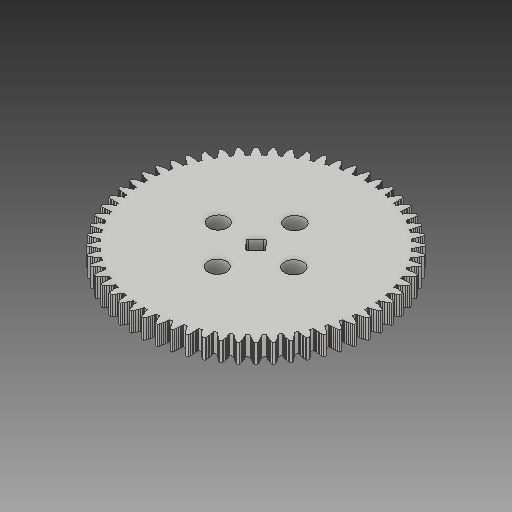
# Autodesk Inventor part: gear60
Saved by Autodesk Inventor 2019 (Build 230136000, 136)
## iProperties
Created: 2019-01-24
Part Number: gear60
Material: Generic
Document SubType Name: Modeling
Designer: Varga Daniel
Density: 1 g/cm^3
Appearance: Default
Author: Varga Daniel
Autodesk Inventor part; units mm, degrees
(part 1 of 2)
ref_plane "YZ Plane" through (0, 0, 0) normal (1, 0, 0) x (0, 1, 0)
ref_plane "XZ Plane" through (0, 0, 0) normal (0, 1, 0) x (-1, 0, 0)
ref_plane "XY Plane" through (0, 0, 0) normal (0, 0, 1) x (1, 0, 0)
sketch "Sketch7" plane through (0, 0, 0) normal (0, 1, 0) x (-1, 0, 0)
  line L0 (2.4527, 31.6296) -> (2.3509, 31.6528)
  line L1 (2.3509, 31.6528) -> (2.2492, 31.6779)
  line L2 (2.2492, 31.6779) -> (2.0459, 31.7329)
  line L3 (2.0459, 31.7329) -> (1.64, 31.8609)
  line L4 (1.64, 31.8609) -> (1.2352, 32.0102)
  line L5 (1.2352, 32.0102) -> (0.8316, 32.1789)
  line L6 (0.8316, 32.1789) -> (0.4294, 32.3655)
  line L7 (0.4294, 32.3655) -> (0.0289, 32.5691)
  line L8 (0.0289, 32.5691) -> (0.0593, 33.1489)
  line L9 (0.0593, 33.1489) -> (0.4789, 33.3096)
  line L10 (0.4789, 33.3096) -> (0.8983, 33.4531)
  line L11 (0.8983, 33.4531) -> (1.3174, 33.5787)
  line L12 (1.3174, 33.5787) -> (1.7356, 33.6849)
  line L13 (1.7356, 33.6849) -> (2.1527, 33.7697)
  line L14 (2.1527, 33.7697) -> (2.3606, 33.8032)
  line L15 (2.3606, 33.8032) -> (2.4644, 33.8175)
  line L16 (2.4644, 33.8175) -> (2.568, 33.83)
  line L17 (2.568, 33.83) -> (2.6526, 34.6349)
  line L18 (2.6526, 34.6349) -> (2.5538, 34.6686)
  line L19 (2.5538, 34.6686) -> (2.4553, 34.7042)
  line L20 (2.4553, 34.7042) -> (2.2589, 34.7802)
  line L21 (2.2589, 34.7802) -> (1.8686, 34.9499)
  line L22 (1.8686, 34.9499) -> (1.4816, 35.1407)
  line L23 (1.4816, 35.1407) -> (1.0978, 35.3506)
  line L24 (1.0978, 35.3506) -> (0.7173, 35.5783)
  line L25 (0.7173, 35.5783) -> (0.3404, 35.8226)
  line L26 (0.3404, 35.8226) -> (0.4312, 36.3961)
  line L27 (0.4312, 36.3961) -> (0.8652, 36.512)
  line L28 (0.8652, 36.512) -> (1.2974, 36.6109)
  line L29 (1.2974, 36.6109) -> (1.7273, 36.692)
  line L30 (1.7273, 36.692) -> (2.1543, 36.7538)
  line L31 (2.1543, 36.7538) -> (2.5779, 36.7946)
  line L32 (2.5779, 36.7946) -> (2.7882, 36.8062)
  line L33 (2.7882, 36.8062) -> (2.8929, 36.8096)
  line L34 (2.8929, 36.8096) -> (2.9973, 36.8112)
  line L35 (2.9973, 36.8112) -> (3.1655, 37.6028)
  line L36 (3.1655, 37.6028) -> (3.0708, 37.6467)
  line L37 (3.0708, 37.6467) -> (2.9766, 37.6924)
  line L38 (2.9766, 37.6924) -> (2.7892, 37.7885)
  line L39 (2.7892, 37.7885) -> (2.4188, 37.998)
  line L40 (2.4188, 37.998) -> (2.0538, 38.2283)
  line L41 (2.0538, 38.2283) -> (1.6941, 38.4772)
  line L42 (1.6941, 38.4772) -> (1.3395, 38.7433)
  line L43 (1.3395, 38.7433) -> (0.9901, 39.0258)
  line L44 (0.9901, 39.0258) -> (1.1404, 39.5866)
  line L45 (1.1404, 39.5866) -> (1.5842, 39.6565)
  line L46 (1.5842, 39.6565) -> (2.0243, 39.7097)
  line L47 (2.0243, 39.7097) -> (2.4603, 39.7454)
  line L48 (2.4603, 39.7454) -> (2.8915, 39.7623)
  line L49 (2.8915, 39.7623) -> (3.3171, 39.7586)
  line L50 (3.3171, 39.7586) -> (3.5274, 39.7481)
  line L51 (3.5274, 39.7481) -> (3.6319, 39.7405)
  line L52 (3.6319, 39.7405) -> (3.7358, 39.7312)
  line L53 (3.7358, 39.7312) -> (3.9859, 40.5009)
  line L54 (3.9859, 40.5009) -> (3.8963, 40.5544)
  line L55 (3.8963, 40.5544) -> (3.8074, 40.6097)
  line L56 (3.8074, 40.6097) -> (3.631, 40.7249)
  line L57 (3.631, 40.7249) -> (3.2846, 40.972)
  line L58 (3.2846, 40.972) -> (2.9457, 41.2391)
  line L59 (2.9457, 41.2391) -> (2.6139, 41.5242)
  line L60 (2.6139, 41.5242) -> (2.2891, 41.826)
  line L61 (2.2891, 41.826) -> (1.9712, 42.1434)
  line L62 (1.9712, 42.1434) -> (2.1792, 42.6854)
  line L63 (2.1792, 42.6854) -> (2.6279, 42.7086)
  line L64 (2.6279, 42.7086) -> (3.0712, 42.7155)
  line L65 (3.0712, 42.7155) -> (3.5085, 42.7054)
  line L66 (3.5085, 42.7054) -> (3.9391, 42.6771)
  line L67 (3.9391, 42.6771) -> (4.362, 42.629)
  line L68 (4.362, 42.629) -> (4.5701, 42.5966)
  line L69 (4.5701, 42.5966) -> (4.6731, 42.5781)
  line L70 (4.6731, 42.5781) -> (4.7756, 42.558)
  line L71 (4.7756, 42.558) -> (5.1047, 43.2973)
  line L72 (5.1047, 43.2973) -> (5.0212, 43.3599)
  line L73 (5.0212, 43.3599) -> (4.9385, 43.4242)
  line L74 (4.9385, 43.4242) -> (4.7752, 43.5572)
  line L75 (4.7752, 43.5572) -> (4.4565, 43.8392)
  line L76 (4.4565, 43.8392) -> (4.1474, 44.1402)
  line L77 (4.1474, 44.1402) -> (3.8472, 44.4585)
  line L78 (3.8472, 44.4585) -> (3.5558, 44.7925)
  line L79 (3.5558, 44.7925) -> (3.2727, 45.1414)
  line L80 (3.2727, 45.1414) -> (3.5363, 45.6588)
  line L81 (3.5363, 45.6588) -> (3.9849, 45.6349)
  line L82 (3.9849, 45.6349) -> (4.4265, 45.5954)
  line L83 (4.4265, 45.5954) -> (4.8604, 45.5397)
  line L84 (4.8604, 45.5397) -> (5.2857, 45.4666)
  line L85 (5.2857, 45.4666) -> (5.7012, 45.3744)
  line L86 (5.7012, 45.3744) -> (5.9047, 45.3205)
  line L87 (5.9047, 45.3205) -> (6.0053, 45.2913)
  line L88 (6.0053, 45.2913) -> (6.1051, 45.2606)
  line L89 (6.1051, 45.2606) -> (6.5097, 45.9615)
  line L90 (6.5097, 45.9615) -> (6.4333, 46.0325)
  line L91 (6.4333, 46.0325) -> (6.3577, 46.105)
  line L92 (6.3577, 46.105) -> (6.2092, 46.2543)
  line L93 (6.2092, 46.2543) -> (5.9217, 46.5681)
  line L94 (5.9217, 46.5681) -> (5.6457, 46.8999)
  line L95 (5.6457, 46.8999) -> (5.3805, 47.2477)
  line L96 (5.3805, 47.2477) -> (5.1255, 47.6104)
  line L97 (5.1255, 47.6104) -> (4.8805, 47.987)
  line L98 (4.8805, 47.987) -> (5.1967, 48.4739)
  line L99 (5.1967, 48.4739) -> (5.6404, 48.4033)
  line L100 (5.6404, 48.4033) -> (6.0755, 48.3179)
  line L101 (6.0755, 48.3179) -> (6.5011, 48.2171)
  line L102 (6.5011, 48.2171) -> (6.9164, 48.0999)
  line L103 (6.9164, 48.0999) -> (7.32, 47.9649)
  line L104 (7.32, 47.9649) -> (7.5168, 47.8899)
  line L105 (7.5168, 47.8899) -> (7.6138, 47.8504)
  line L106 (7.6138, 47.8504) -> (7.7098, 47.8094)
  line L107 (7.7098, 47.8094) -> (8.1855, 48.4642)
  line L108 (8.1855, 48.4642) -> (8.1169, 48.5428)
  line L109 (8.1169, 48.5428) -> (8.0493, 48.6228)
  line L110 (8.0493, 48.6228) -> (7.9172, 48.7869)
  line L111 (7.9172, 48.7869) -> (7.6641, 49.129)
  line L112 (7.6641, 49.129) -> (7.4243, 49.4878)
  line L113 (7.4243, 49.4878) -> (7.1969, 49.8614)
  line L114 (7.1969, 49.8614) -> (6.9813, 50.2488)
  line L115 (6.9813, 50.2488) -> (6.777, 50.6489)
  line L116 (6.777, 50.6489) -> (7.1423, 51.1001)
  line L117 (7.1423, 51.1001) -> (7.5762, 50.9835)
  line L118 (7.5762, 50.9835) -> (7.9999, 50.8531)
  line L119 (7.9999, 50.8531) -> (8.4127, 50.7084)
  line L120 (8.4127, 50.7084) -> (8.8135, 50.5484)
  line L121 (8.8135, 50.5484) -> (9.2008, 50.3719)
  line L122 (9.2008, 50.3719) -> (9.3887, 50.2768)
  line L123 (9.3887, 50.2768) -> (9.481, 50.2274)
  line L124 (9.481, 50.2274) -> (9.5722, 50.1766)
  line L125 (9.5722, 50.1766) -> (10.1137, 50.778)
  line L126 (10.1137, 50.778) -> (10.0537, 50.8634)
  line L127 (10.0537, 50.8634) -> (9.9948, 50.9501)
  line L128 (9.9948, 50.9501) -> (9.8806, 51.127)
  line L129 (9.8806, 51.127) -> (9.6646, 51.4937)
  line L130 (9.6646, 51.4937) -> (9.4637, 51.8755)
  line L131 (9.4637, 51.8755) -> (9.2766, 52.2709)
  line L132 (9.2766, 52.2709) -> (9.1026, 52.6787)
  line L133 (9.1026, 52.6787) -> (8.9413, 53.098)
  line L134 (8.9413, 53.098) -> (9.3518, 53.5086)
  line L135 (9.3518, 53.5086) -> (9.7711, 53.3472)
  line L136 (9.7711, 53.3472) -> (10.1789, 53.1732)
  line L137 (10.1789, 53.1732) -> (10.5743, 52.9861)
  line L138 (10.5743, 52.9861) -> (10.9561, 52.7852)
  line L139 (10.9561, 52.7852) -> (11.3228, 52.5692)
  line L140 (11.3228, 52.5692) -> (11.4998, 52.455)
  line L141 (11.4998, 52.455) -> (11.5864, 52.3961)
  line L142 (11.5864, 52.3961) -> (11.6718, 52.3361)
  line L143 (11.6718, 52.3361) -> (12.2732, 52.8776)
  line L144 (12.2732, 52.8776) -> (12.2224, 52.9688)
  line L145 (12.2224, 52.9688) -> (12.173, 53.0611)
  line L146 (12.173, 53.0611) -> (12.0779, 53.249)
  line L147 (12.0779, 53.249) -> (11.9014, 53.6363)
  line L148 (11.9014, 53.6363) -> (11.7415, 54.0371)
  line L149 (11.7415, 54.0371) -> (11.5967, 54.4499)
  line L150 (11.5967, 54.4499) -> (11.4663, 54.8736)
  line L151 (11.4663, 54.8736) -> (11.3497, 55.3075)
  line L152 (11.3497, 55.3075) -> (11.8009, 55.6728)
  line L153 (11.8009, 55.6728) -> (12.201, 55.4686)
  line L154 (12.201, 55.4686) -> (12.5884, 55.2529)
  line L155 (12.5884, 55.2529) -> (12.9621, 55.0255)
  line L156 (12.9621, 55.0255) -> (13.3208, 54.7857)
  line L157 (13.3208, 54.7857) -> (13.663, 54.5326)
  line L158 (13.663, 54.5326) -> (13.827, 54.4005)
  line L159 (13.827, 54.4005) -> (13.907, 54.3329)
  line L160 (13.907, 54.3329) -> (13.9856, 54.2643)
  line L161 (13.9856, 54.2643) -> (14.6404, 54.74)
  line L162 (14.6404, 54.74) -> (14.5994, 54.836)
  line L163 (14.5994, 54.836) -> (14.5599, 54.933)
  line L164 (14.5599, 54.933) -> (14.4849, 55.1298)
  line L165 (14.4849, 55.1298) -> (14.3499, 55.5334)
  line L166 (14.3499, 55.5334) -> (14.2327, 55.9487)
  line L167 (14.2327, 55.9487) -> (14.1319, 56.3743)
  line L168 (14.1319, 56.3743) -> (14.0465, 56.8094)
  line L169 (14.0465, 56.8094) -> (13.9759, 57.2531)
  line L170 (13.9759, 57.2531) -> (14.4628, 57.5693)
  line L171 (14.4628, 57.5693) -> (14.8394, 57.3243)
  line L172 (14.8394, 57.3243) -> (15.2021, 57.0693)
  line L173 (15.2021, 57.0693) -> (15.55, 56.8041)
  line L174 (15.55, 56.8041) -> (15.8817, 56.5282)
  line L175 (15.8817, 56.5282) -> (16.1955, 56.2406)
  line L176 (16.1955, 56.2406) -> (16.3448, 56.0921)
  line L177 (16.3448, 56.0921) -> (16.4173, 56.0166)
  line L178 (16.4173, 56.0166) -> (16.4883, 55.9401)
  line L179 (16.4883, 55.9401) -> (17.1892, 56.3447)
  line L180 (17.1892, 56.3447) -> (17.1585, 56.4445)
  line L181 (17.1585, 56.4445) -> (17.1293, 56.5451)
  line L182 (17.1293, 56.5451) -> (17.0754, 56.7486)
  line L183 (17.0754, 56.7486) -> (16.9833, 57.1642)
  line L184 (16.9833, 57.1642) -> (16.9101, 57.5894)
  line L185 (16.9101, 57.5894) -> (16.8544, 58.0233)
  line L186 (16.8544, 58.0233) -> (16.8149, 58.4649)
  line L187 (16.8149, 58.4649) -> (16.7911, 58.9135)
  line L188 (16.7911, 58.9135) -> (17.3084, 59.1771)
  line L189 (17.3084, 59.1771) -> (17.6573, 58.8941)
  line L190 (17.6573, 58.8941) -> (17.9913, 58.6026)
  line L191 (17.9913, 58.6026) -> (18.3096, 58.3025)
  line L192 (18.3096, 58.3025) -> (18.6106, 57.9933)
  line L193 (18.6106, 57.9933) -> (18.8927, 57.6746)
  line L194 (18.8927, 57.6746) -> (19.0256, 57.5113)
  line L195 (19.0256, 57.5113) -> (19.0899, 57.4286)
  line L196 (19.0899, 57.4286) -> (19.1525, 57.3451)
  line L197 (19.1525, 57.3451) -> (19.8919, 57.6743)
  line L198 (19.8919, 57.6743) -> (19.8717, 57.7767)
  line L199 (19.8717, 57.7767) -> (19.8532, 57.8798)
  line L200 (19.8532, 57.8798) -> (19.8208, 58.0879)
  line L201 (19.8208, 58.0879) -> (19.7727, 58.5107)
  line L202 (19.7727, 58.5107) -> (19.7444, 58.9413)
  line L203 (19.7444, 58.9413) -> (19.7343, 59.3786)
  line L204 (19.7343, 59.3786) -> (19.7412, 59.8219)
  line L205 (19.7412, 59.8219) -> (19.7644, 60.2706)
  line L206 (19.7644, 60.2706) -> (20.3064, 60.4786)
  line L207 (20.3064, 60.4786) -> (20.6238, 60.1607)
  line L208 (20.6238, 60.1607) -> (20.9256, 59.8359)
  line L209 (20.9256, 59.8359) -> (21.2107, 59.5042)
  line L210 (21.2107, 59.5042) -> (21.4778, 59.1653)
  line L211 (21.4778, 59.1653) -> (21.725, 58.8188)
  line L212 (21.725, 58.8188) -> (21.8401, 58.6425)
  line L213 (21.8401, 58.6425) -> (21.8954, 58.5535)
  line L214 (21.8954, 58.5535) -> (21.949, 58.4639)
  line L215 (21.949, 58.4639) -> (22.7186, 58.714)
  line L216 (22.7186, 58.714) -> (22.7093, 58.8179)
  line L217 (22.7093, 58.8179) -> (22.7017, 58.9224)
  line L218 (22.7017, 58.9224) -> (22.6913, 59.1327)
  line L219 (22.6913, 59.1327) -> (22.6876, 59.5583)
  line L220 (22.6876, 59.5583) -> (22.7045, 59.9895)
  line L221 (22.7045, 59.9895) -> (22.7401, 60.4255)
  line L222 (22.7401, 60.4255) -> (22.7933, 60.8656)
  line L223 (22.7933, 60.8656) -> (22.8633, 61.3094)
  line L224 (22.8633, 61.3094) -> (23.4241, 61.4597)
  line L225 (23.4241, 61.4597) -> (23.7065, 61.1103)
  line L226 (23.7065, 61.1103) -> (23.9727, 60.7557)
  line L227 (23.9727, 60.7557) -> (24.2216, 60.396)
  line L228 (24.2216, 60.396) -> (24.4518, 60.031)
  line L229 (24.4518, 60.031) -> (24.6613, 59.6606)
  line L230 (24.6613, 59.6606) -> (24.7575, 59.4733)
  line L231 (24.7575, 59.4733) -> (24.8031, 59.379)
  line L232 (24.8031, 59.379) -> (24.847, 59.2843)
  line L233 (24.847, 59.2843) -> (25.6386, 59.4525)
  line L234 (25.6386, 59.4525) -> (25.6402, 59.5569)
  line L235 (25.6402, 59.5569) -> (25.6436, 59.6616)
  line L236 (25.6436, 59.6616) -> (25.6552, 59.8719)
  line L237 (25.6552, 59.8719) -> (25.696, 60.2955)
  line L238 (25.696, 60.2955) -> (25.7578, 60.7225)
  line L239 (25.7578, 60.7225) -> (25.8389, 61.1524)
  line L240 (25.8389, 61.1524) -> (25.9378, 61.5846)
  line L241 (25.9378, 61.5846) -> (26.0538, 62.0186)
  line L242 (26.0538, 62.0186) -> (26.6272, 62.1095)
  line L243 (26.6272, 62.1095) -> (26.8716, 61.7325)
  line L244 (26.8716, 61.7325) -> (27.0992, 61.352)
  line L245 (27.0992, 61.352) -> (27.3091, 60.9682)
  line L246 (27.3091, 60.9682) -> (27.4999, 60.5812)
  line L247 (27.4999, 60.5812) -> (27.6697, 60.1909)
  line L248 (27.6697, 60.1909) -> (27.7456, 59.9945)
  line L249 (27.7456, 59.9945) -> (27.7812, 59.896)
  line L250 (27.7812, 59.896) -> (27.8149, 59.7972)
  line L251 (27.8149, 59.7972) -> (28.6198, 59.8818)
  line L252 (28.6198, 59.8818) -> (28.6323, 59.9855)
  line L253 (28.6323, 59.9855) -> (28.6466, 60.0892)
  line L254 (28.6466, 60.0892) -> (28.6801, 60.2971)
  line L255 (28.6801, 60.2971) -> (28.765, 60.7142)
  line L256 (28.765, 60.7142) -> (28.8711, 61.1324)
  line L257 (28.8711, 61.1324) -> (28.9967, 61.5515)
  line L258 (28.9967, 61.5515) -> (29.1403, 61.9709)
  line L259 (29.1403, 61.9709) -> (29.3009, 62.3905)
  line L260 (29.3009, 62.3905) -> (29.8807, 62.4209)
  line L261 (29.8807, 62.4209) -> (30.0843, 62.0204)
  line L262 (30.0843, 62.0204) -> (30.2709, 61.6182)
  line L263 (30.2709, 61.6182) -> (30.4396, 61.2146)
  line L264 (30.4396, 61.2146) -> (30.5889, 60.8098)
  line L265 (30.5889, 60.8098) -> (30.7169, 60.4039)
  line L266 (30.7169, 60.4039) -> (30.772, 60.2006)
  line L267 (30.772, 60.2006) -> (30.797, 60.0989)
  line L268 (30.797, 60.0989) -> (30.8203, 59.9972)
  line L269 (30.8203, 59.9972) -> (31.6296, 59.9972)
  line L270 (31.6296, 59.9972) -> (31.6528, 60.0989)
  line L271 (31.6528, 60.0989) -> (31.6779, 60.2006)
  line L272 (31.6779, 60.2006) -> (31.7329, 60.4039)
  line L273 (31.7329, 60.4039) -> (31.8609, 60.8098)
  line L274 (31.8609, 60.8098) -> (32.0102, 61.2146)
  line L275 (32.0102, 61.2146) -> (32.1789, 61.6182)
  line L276 (32.1789, 61.6182) -> (32.3655, 62.0204)
  line L277 (32.3655, 62.0204) -> (32.5691, 62.4209)
  line L278 (32.5691, 62.4209) -> (33.1489, 62.3905)
  line L279 (33.1489, 62.3905) -> (33.3096, 61.9709)
  line L280 (33.3096, 61.9709) -> (33.4531, 61.5515)
  line L281 (33.4531, 61.5515) -> (33.5787, 61.1324)
  line L282 (33.5787, 61.1324) -> (33.6849, 60.7142)
  line L283 (33.6849, 60.7142) -> (33.7697, 60.2971)
  line L284 (33.7697, 60.2971) -> (33.8032, 60.0892)
  line L285 (33.8032, 60.0892) -> (33.8175, 59.9855)
  line L286 (33.8175, 59.9855) -> (33.83, 59.8818)
  line L287 (33.83, 59.8818) -> (34.6349, 59.7972)
  line L288 (34.6349, 59.7972) -> (34.6686, 59.896)
  line L289 (34.6686, 59.896) -> (34.7042, 59.9945)
  line L290 (34.7042, 59.9945) -> (34.7802, 60.1909)
  line L291 (34.7802, 60.1909) -> (34.9499, 60.5812)
  line L292 (34.9499, 60.5812) -> (35.1407, 60.9682)
  line L293 (35.1407, 60.9682) -> (35.3506, 61.352)
  line L294 (35.3506, 61.352) -> (35.5783, 61.7325)
  line L295 (35.5783, 61.7325) -> (35.8226, 62.1095)
  line L296 (35.8226, 62.1095) -> (36.3961, 62.0186)
  line L297 (36.3961, 62.0186) -> (36.512, 61.5846)
  line L298 (36.512, 61.5846) -> (36.6109, 61.1524)
  line L299 (36.6109, 61.1524) -> (36.692, 60.7225)
  line L300 (36.692, 60.7225) -> (36.7538, 60.2955)
  line L301 (36.7538, 60.2955) -> (36.7946, 59.8719)
  line L302 (36.7946, 59.8719) -> (36.8062, 59.6616)
  line L303 (36.8062, 59.6616) -> (36.8096, 59.5569)
  line L304 (36.8096, 59.5569) -> (36.8112, 59.4525)
  line L305 (36.8112, 59.4525) -> (37.6028, 59.2843)
  line L306 (37.6028, 59.2843) -> (37.6467, 59.379)
  line L307 (37.6467, 59.379) -> (37.6924, 59.4733)
  line L308 (37.6924, 59.4733) -> (37.7885, 59.6606)
  line L309 (37.7885, 59.6606) -> (37.998, 60.031)
  line L310 (37.998, 60.031) -> (38.2283, 60.396)
  line L311 (38.2283, 60.396) -> (38.4772, 60.7557)
  line L312 (38.4772, 60.7557) -> (38.7433, 61.1103)
  line L313 (38.7433, 61.1103) -> (39.0258, 61.4597)
  line L314 (39.0258, 61.4597) -> (39.5866, 61.3094)
  line L315 (39.5866, 61.3094) -> (39.6565, 60.8656)
  line L316 (39.6565, 60.8656) -> (39.7097, 60.4255)
  line L317 (39.7097, 60.4255) -> (39.7454, 59.9895)
  line L318 (39.7454, 59.9895) -> (39.7623, 59.5583)
  line L319 (39.7623, 59.5583) -> (39.7586, 59.1327)
  line L320 (39.7586, 59.1327) -> (39.7481, 58.9224)
  line L321 (39.7481, 58.9224) -> (39.7405, 58.8179)
  line L322 (39.7405, 58.8179) -> (39.7312, 58.714)
  line L323 (39.7312, 58.714) -> (40.5009, 58.4639)
  line L324 (40.5009, 58.4639) -> (40.5544, 58.5535)
  line L325 (40.5544, 58.5535) -> (40.6097, 58.6425)
  line L326 (40.6097, 58.6425) -> (40.7249, 58.8188)
  line L327 (40.7249, 58.8188) -> (40.972, 59.1653)
  line L328 (40.972, 59.1653) -> (41.2391, 59.5042)
  line L329 (41.2391, 59.5042) -> (41.5242, 59.8359)
  line L330 (41.5242, 59.8359) -> (41.826, 60.1607)
  line L331 (41.826, 60.1607) -> (42.1434, 60.4786)
  line L332 (42.1434, 60.4786) -> (42.6854, 60.2706)
  line L333 (42.6854, 60.2706) -> (42.7086, 59.8219)
  line L334 (42.7086, 59.8219) -> (42.7155, 59.3786)
  line L335 (42.7155, 59.3786) -> (42.7054, 58.9413)
  line L336 (42.7054, 58.9413) -> (42.6771, 58.5107)
  line L337 (42.6771, 58.5107) -> (42.629, 58.0879)
  line L338 (42.629, 58.0879) -> (42.5966, 57.8798)
  line L339 (42.5966, 57.8798) -> (42.5781, 57.7767)
  line L340 (42.5781, 57.7767) -> (42.558, 57.6743)
  line L341 (42.558, 57.6743) -> (43.2973, 57.3451)
  line L342 (43.2973, 57.3451) -> (43.3599, 57.4286)
  line L343 (43.3599, 57.4286) -> (43.4242, 57.5113)
  line L344 (43.4242, 57.5113) -> (43.5572, 57.6746)
  line L345 (43.5572, 57.6746) -> (43.8392, 57.9933)
  line L346 (43.8392, 57.9933) -> (44.1402, 58.3025)
  line L347 (44.1402, 58.3025) -> (44.4585, 58.6026)
  line L348 (44.4585, 58.6026) -> (44.7925, 58.8941)
  line L349 (44.7925, 58.8941) -> (45.1414, 59.1771)
  line L350 (45.1414, 59.1771) -> (45.6588, 58.9135)
  line L351 (45.6588, 58.9135) -> (45.6349, 58.4649)
  line L352 (45.6349, 58.4649) -> (45.5954, 58.0233)
  line L353 (45.5954, 58.0233) -> (45.5397, 57.5894)
  line L354 (45.5397, 57.5894) -> (45.4666, 57.1642)
  line L355 (45.4666, 57.1642) -> (45.3744, 56.7486)
  line L356 (45.3744, 56.7486) -> (45.3205, 56.5451)
  line L357 (45.3205, 56.5451) -> (45.2913, 56.4445)
  line L358 (45.2913, 56.4445) -> (45.2606, 56.3447)
  line L359 (45.2606, 56.3447) -> (45.9615, 55.9401)
  line L360 (45.9615, 55.9401) -> (46.0325, 56.0166)
  line L361 (46.0325, 56.0166) -> (46.105, 56.0921)
  line L362 (46.105, 56.0921) -> (46.2543, 56.2406)
  line L363 (46.2543, 56.2406) -> (46.5681, 56.5282)
  line L364 (46.5681, 56.5282) -> (46.8999, 56.8041)
  line L365 (46.8999, 56.8041) -> (47.2477, 57.0693)
  line L366 (47.2477, 57.0693) -> (47.6104, 57.3243)
  line L367 (47.6104, 57.3243) -> (47.987, 57.5693)
  line L368 (47.987, 57.5693) -> (48.4739, 57.2531)
  line L369 (48.4739, 57.2531) -> (48.4033, 56.8094)
  line L370 (48.4033, 56.8094) -> (48.3179, 56.3743)
  line L371 (48.3179, 56.3743) -> (48.2171, 55.9487)
  line L372 (48.2171, 55.9487) -> (48.0999, 55.5334)
  line L373 (48.0999, 55.5334) -> (47.9649, 55.1298)
  line L374 (47.9649, 55.1298) -> (47.8899, 54.933)
  line L375 (47.8899, 54.933) -> (47.8504, 54.836)
  line L376 (47.8504, 54.836) -> (47.8094, 54.74)
  line L377 (47.8094, 54.74) -> (48.4642, 54.2643)
  line L378 (48.4642, 54.2643) -> (48.5428, 54.3329)
  line L379 (48.5428, 54.3329) -> (48.6228, 54.4005)
  line L380 (48.6228, 54.4005) -> (48.7869, 54.5326)
  line L381 (48.7869, 54.5326) -> (49.129, 54.7857)
  line L382 (49.129, 54.7857) -> (49.4878, 55.0255)
  line L383 (49.4878, 55.0255) -> (49.8614, 55.2529)
  line L384 (49.8614, 55.2529) -> (50.2488, 55.4686)
  line L385 (50.2488, 55.4686) -> (50.6489, 55.6728)
  line L386 (50.6489, 55.6728) -> (51.1001, 55.3075)
  line L387 (51.1001, 55.3075) -> (50.9835, 54.8736)
  line L388 (50.9835, 54.8736) -> (50.8531, 54.4499)
  line L389 (50.8531, 54.4499) -> (50.7084, 54.0371)
  line L390 (50.7084, 54.0371) -> (50.5484, 53.6363)
  line L391 (50.5484, 53.6363) -> (50.3719, 53.249)
  line L392 (50.3719, 53.249) -> (50.2768, 53.0611)
  line L393 (50.2768, 53.0611) -> (50.2274, 52.9688)
  line L394 (50.2274, 52.9688) -> (50.1766, 52.8776)
  line L395 (50.1766, 52.8776) -> (50.778, 52.3361)
  line L396 (50.778, 52.3361) -> (50.8634, 52.3961)
  line L397 (50.8634, 52.3961) -> (50.9501, 52.455)
  line L398 (50.9501, 52.455) -> (51.127, 52.5692)
  line L399 (51.127, 52.5692) -> (51.4937, 52.7852)
  line L400 (51.4937, 52.7852) -> (51.8755, 52.9861)
  line L401 (51.8755, 52.9861) -> (52.2709, 53.1732)
  line L402 (52.2709, 53.1732) -> (52.6787, 53.3472)
  line L403 (52.6787, 53.3472) -> (53.098, 53.5086)
  line L404 (53.098, 53.5086) -> (53.5086, 53.098)
  line L405 (53.5086, 53.098) -> (53.3472, 52.6787)
  line L406 (53.3472, 52.6787) -> (53.1732, 52.2709)
  line L407 (53.1732, 52.2709) -> (52.9861, 51.8755)
  line L408 (52.9861, 51.8755) -> (52.7852, 51.4937)
  line L409 (52.7852, 51.4937) -> (52.5692, 51.127)
  line L410 (52.5692, 51.127) -> (52.455, 50.9501)
  line L411 (52.455, 50.9501) -> (52.3961, 50.8634)
  line L412 (52.3961, 50.8634) -> (52.3361, 50.778)
  line L413 (52.3361, 50.778) -> (52.8776, 50.1766)
  line L414 (52.8776, 50.1766) -> (52.9688, 50.2274)
  line L415 (52.9688, 50.2274) -> (53.0611, 50.2768)
  line L416 (53.0611, 50.2768) -> (53.249, 50.3719)
  line L417 (53.249, 50.3719) -> (53.6363, 50.5484)
  line L418 (53.6363, 50.5484) -> (54.0371, 50.7084)
  line L419 (54.0371, 50.7084) -> (54.4499, 50.8531)
  line L420 (54.4499, 50.8531) -> (54.8736, 50.9835)
  line L421 (54.8736, 50.9835) -> (55.3075, 51.1001)
  line L422 (55.3075, 51.1001) -> (55.6728, 50.6489)
  line L423 (55.6728, 50.6489) -> (55.4686, 50.2488)
  line L424 (55.4686, 50.2488) -> (55.2529, 49.8614)
  line L425 (55.2529, 49.8614) -> (55.0255, 49.4878)
  line L426 (55.0255, 49.4878) -> (54.7857, 49.129)
  line L427 (54.7857, 49.129) -> (54.5326, 48.7869)
  line L428 (54.5326, 48.7869) -> (54.4005, 48.6228)
  line L429 (54.4005, 48.6228) -> (54.3329, 48.5428)
  line L430 (54.3329, 48.5428) -> (54.2643, 48.4642)
  line L431 (54.2643, 48.4642) -> (54.74, 47.8094)
  line L432 (54.74, 47.8094) -> (54.836, 47.8504)
  line L433 (54.836, 47.8504) -> (54.933, 47.8899)
  line L434 (54.933, 47.8899) -> (55.1298, 47.9649)
  line L435 (55.1298, 47.9649) -> (55.5334, 48.0999)
  line L436 (55.5334, 48.0999) -> (55.9487, 48.2171)
  line L437 (55.9487, 48.2171) -> (56.3743, 48.3179)
  line L438 (56.3743, 48.3179) -> (56.8094, 48.4033)
  line L439 (56.8094, 48.4033) -> (57.2531, 48.4739)
  line L440 (57.2531, 48.4739) -> (57.5693, 47.987)
  line L441 (57.5693, 47.987) -> (57.3243, 47.6104)
  line L442 (57.3243, 47.6104) -> (57.0693, 47.2477)
  line L443 (57.0693, 47.2477) -> (56.8041, 46.8999)
  line L444 (56.8041, 46.8999) -> (56.5282, 46.5681)
  line L445 (56.5282, 46.5681) -> (56.2406, 46.2543)
  line L446 (56.2406, 46.2543) -> (56.0921, 46.105)
  line L447 (56.0921, 46.105) -> (56.0166, 46.0325)
  line L448 (56.0166, 46.0325) -> (55.9401, 45.9615)
  line L449 (55.9401, 45.9615) -> (56.3447, 45.2606)
  line L450 (56.3447, 45.2606) -> (56.4445, 45.2913)
  line L451 (56.4445, 45.2913) -> (56.5451, 45.3205)
  line L452 (56.5451, 45.3205) -> (56.7486, 45.3744)
  line L453 (56.7486, 45.3744) -> (57.1642, 45.4666)
  line L454 (57.1642, 45.4666) -> (57.5894, 45.5397)
  line L455 (57.5894, 45.5397) -> (58.0233, 45.5954)
  line L456 (58.0233, 45.5954) -> (58.4649, 45.6349)
  line L457 (58.4649, 45.6349) -> (58.9135, 45.6588)
  line L458 (58.9135, 45.6588) -> (59.1771, 45.1414)
  line L459 (59.1771, 45.1414) -> (58.8941, 44.7925)
  line L460 (58.8941, 44.7925) -> (58.6026, 44.4585)
  line L461 (58.6026, 44.4585) -> (58.3025, 44.1402)
  line L462 (58.3025, 44.1402) -> (57.9933, 43.8392)
  line L463 (57.9933, 43.8392) -> (57.6746, 43.5572)
  line L464 (57.6746, 43.5572) -> (57.5113, 43.4242)
  line L465 (57.5113, 43.4242) -> (57.4286, 43.3599)
  line L466 (57.4286, 43.3599) -> (57.3451, 43.2973)
  line L467 (57.3451, 43.2973) -> (57.6743, 42.558)
  line L468 (57.6743, 42.558) -> (57.7767, 42.5781)
  line L469 (57.7767, 42.5781) -> (57.8798, 42.5966)
  line L470 (57.8798, 42.5966) -> (58.0879, 42.629)
  line L471 (58.0879, 42.629) -> (58.5107, 42.6771)
  line L472 (58.5107, 42.6771) -> (58.9413, 42.7054)
  line L473 (58.9413, 42.7054) -> (59.3786, 42.7155)
  line L474 (59.3786, 42.7155) -> (59.8219, 42.7086)
  line L475 (59.8219, 42.7086) -> (60.2706, 42.6854)
  line L476 (60.2706, 42.6854) -> (60.4786, 42.1434)
  line L477 (60.4786, 42.1434) -> (60.1607, 41.826)
  line L478 (60.1607, 41.826) -> (59.8359, 41.5242)
  line L479 (59.8359, 41.5242) -> (59.5042, 41.2391)
  line L480 (59.5042, 41.2391) -> (59.1653, 40.972)
  line L481 (59.1653, 40.972) -> (58.8188, 40.7249)
  line L482 (58.8188, 40.7249) -> (58.6425, 40.6097)
  line L483 (58.6425, 40.6097) -> (58.5535, 40.5544)
  line L484 (58.5535, 40.5544) -> (58.4639, 40.5009)
  line L485 (58.4639, 40.5009) -> (58.714, 39.7312)
  line L486 (58.714, 39.7312) -> (58.8179, 39.7405)
  line L487 (58.8179, 39.7405) -> (58.9224, 39.7481)
  line L488 (58.9224, 39.7481) -> (59.1327, 39.7586)
  line L489 (59.1327, 39.7586) -> (59.5583, 39.7623)
  line L490 (59.5583, 39.7623) -> (59.9895, 39.7454)
  line L491 (59.9895, 39.7454) -> (60.4255, 39.7097)
  line L492 (60.4255, 39.7097) -> (60.8656, 39.6565)
  line L493 (60.8656, 39.6565) -> (61.3094, 39.5866)
  line L494 (61.3094, 39.5866) -> (61.4597, 39.0258)
  line L495 (61.4597, 39.0258) -> (61.1103, 38.7433)
  line L496 (61.1103, 38.7433) -> (60.7557, 38.4772)
  line L497 (60.7557, 38.4772) -> (60.396, 38.2283)
  line L498 (60.396, 38.2283) -> (60.031, 37.998)
  line L499 (60.031, 37.998) -> (59.6606, 37.7885)
  line L500 (59.6606, 37.7885) -> (59.4733, 37.6924)
  line L501 (59.4733, 37.6924) -> (59.379, 37.6467)
  line L502 (59.379, 37.6467) -> (59.2843, 37.6028)
  line L503 (59.2843, 37.6028) -> (59.4525, 36.8112)
  line L504 (59.4525, 36.8112) -> (59.5569, 36.8096)
  line L505 (59.5569, 36.8096) -> (59.6616, 36.8062)
  line L506 (59.6616, 36.8062) -> (59.8719, 36.7946)
  line L507 (59.8719, 36.7946) -> (60.2955, 36.7538)
  line L508 (60.2955, 36.7538) -> (60.7225, 36.692)
  line L509 (60.7225, 36.692) -> (61.1524, 36.6109)
  line L510 (61.1524, 36.6109) -> (61.5846, 36.512)
  line L511 (61.5846, 36.512) -> (62.0186, 36.3961)
  line L512 (62.0186, 36.3961) -> (62.1095, 35.8226)
  line L513 (62.1095, 35.8226) -> (61.7325, 35.5783)
  line L514 (61.7325, 35.5783) -> (61.352, 35.3506)
  line L515 (61.352, 35.3506) -> (60.9682, 35.1407)
  line L516 (60.9682, 35.1407) -> (60.5812, 34.9499)
  line L517 (60.5812, 34.9499) -> (60.1909, 34.7802)
  line L518 (60.1909, 34.7802) -> (59.9945, 34.7042)
  line L519 (59.9945, 34.7042) -> (59.896, 34.6686)
  line L520 (59.896, 34.6686) -> (59.7972, 34.6349)
  line L521 (59.7972, 34.6349) -> (59.8818, 33.83)
  line L522 (59.8818, 33.83) -> (59.9855, 33.8175)
  line L523 (59.9855, 33.8175) -> (60.0892, 33.8032)
  line L524 (60.0892, 33.8032) -> (60.2971, 33.7697)
  line L525 (60.2971, 33.7697) -> (60.7142, 33.6849)
  line L526 (60.7142, 33.6849) -> (61.1324, 33.5787)
  line L527 (61.1324, 33.5787) -> (61.5515, 33.4531)
  line L528 (61.5515, 33.4531) -> (61.9709, 33.3096)
  line L529 (61.9709, 33.3096) -> (62.3905, 33.1489)
  line L530 (62.3905, 33.1489) -> (62.4209, 32.5691)
  line L531 (62.4209, 32.5691) -> (62.0204, 32.3655)
  line L532 (62.0204, 32.3655) -> (61.6182, 32.1789)
  line L533 (61.6182, 32.1789) -> (61.2146, 32.0102)
  line L534 (61.2146, 32.0102) -> (60.8098, 31.8609)
  line L535 (60.8098, 31.8609) -> (60.4039, 31.7329)
  line L536 (60.4039, 31.7329) -> (60.2006, 31.6779)
  line L537 (60.2006, 31.6779) -> (60.0989, 31.6528)
  line L538 (60.0989, 31.6528) -> (59.9972, 31.6296)
  line L539 (59.9972, 31.6296) -> (59.9972, 30.8203)
  line L540 (59.9972, 30.8203) -> (60.0989, 30.797)
  line L541 (60.0989, 30.797) -> (60.2006, 30.772)
  line L542 (60.2006, 30.772) -> (60.4039, 30.7169)
  line L543 (60.4039, 30.7169) -> (60.8098, 30.5889)
  line L544 (60.8098, 30.5889) -> (61.2146, 30.4396)
  line L545 (61.2146, 30.4396) -> (61.6182, 30.2709)
  line L546 (61.6182, 30.2709) -> (62.0204, 30.0843)
  line L547 (62.0204, 30.0843) -> (62.4209, 29.8807)
  line L548 (62.4209, 29.8807) -> (62.3905, 29.3009)
  line L549 (62.3905, 29.3009) -> (61.9709, 29.1403)
  line L550 (61.9709, 29.1403) -> (61.5515, 28.9967)
  line L551 (61.5515, 28.9967) -> (61.1324, 28.8711)
  line L552 (61.1324, 28.8711) -> (60.7142, 28.765)
  line L553 (60.7142, 28.765) -> (60.2971, 28.6801)
  line L554 (60.2971, 28.6801) -> (60.0892, 28.6466)
  line L555 (60.0892, 28.6466) -> (59.9855, 28.6323)
  line L556 (59.9855, 28.6323) -> (59.8818, 28.6198)
  line L557 (59.8818, 28.6198) -> (59.7972, 27.8149)
  line L558 (59.7972, 27.8149) -> (59.896, 27.7812)
  line L559 (59.896, 27.7812) -> (59.9945, 27.7456)
  line L560 (59.9945, 27.7456) -> (60.1909, 27.6697)
  line L561 (60.1909, 27.6697) -> (60.5812, 27.4999)
  line L562 (60.5812, 27.4999) -> (60.9682, 27.3091)
  line L563 (60.9682, 27.3091) -> (61.352, 27.0992)
  line L564 (61.352, 27.0992) -> (61.7325, 26.8716)
  line L565 (61.7325, 26.8716) -> (62.1095, 26.6272)
  line L566 (62.1095, 26.6272) -> (62.0186, 26.0538)
  line L567 (62.0186, 26.0538) -> (61.5846, 25.9378)
  line L568 (61.5846, 25.9378) -> (61.1524, 25.8389)
  line L569 (61.1524, 25.8389) -> (60.7225, 25.7578)
  line L570 (60.7225, 25.7578) -> (60.2955, 25.696)
  line L571 (60.2955, 25.696) -> (59.8719, 25.6552)
  line L572 (59.8719, 25.6552) -> (59.6616, 25.6436)
  line L573 (59.6616, 25.6436) -> (59.5569, 25.6402)
  line L574 (59.5569, 25.6402) -> (59.4525, 25.6386)
  line L575 (59.4525, 25.6386) -> (59.2843, 24.847)
  line L576 (59.2843, 24.847) -> (59.379, 24.8031)
  line L577 (59.379, 24.8031) -> (59.4733, 24.7575)
  line L578 (59.4733, 24.7575) -> (59.6606, 24.6613)
  line L579 (59.6606, 24.6613) -> (60.031, 24.4518)
  line L580 (60.031, 24.4518) -> (60.396, 24.2216)
  line L581 (60.396, 24.2216) -> (60.7557, 23.9727)
  line L582 (60.7557, 23.9727) -> (61.1103, 23.7065)
  line L583 (61.1103, 23.7065) -> (61.4597, 23.4241)
  line L584 (61.4597, 23.4241) -> (61.3094, 22.8633)
  line L585 (61.3094, 22.8633) -> (60.8656, 22.7933)
  line L586 (60.8656, 22.7933) -> (60.4255, 22.7401)
  line L587 (60.4255, 22.7401) -> (59.9895, 22.7045)
  line L588 (59.9895, 22.7045) -> (59.5583, 22.6876)
  line L589 (59.5583, 22.6876) -> (59.1327, 22.6913)
  line L590 (59.1327, 22.6913) -> (58.9224, 22.7017)
  line L591 (58.9224, 22.7017) -> (58.8179, 22.7093)
  line L592 (58.8179, 22.7093) -> (58.714, 22.7186)
  line L593 (58.714, 22.7186) -> (58.4639, 21.949)
  line L594 (58.4639, 21.949) -> (58.5535, 21.8954)
  line L595 (58.5535, 21.8954) -> (58.6425, 21.8401)
  line L596 (58.6425, 21.8401) -> (58.8188, 21.725)
  line L597 (58.8188, 21.725) -> (59.1653, 21.4778)
  line L598 (59.1653, 21.4778) -> (59.5042, 21.2107)
  line L599 (59.5042, 21.2107) -> (59.8359, 20.9256)
  line L600 (59.8359, 20.9256) -> (60.1607, 20.6238)
  line L601 (60.1607, 20.6238) -> (60.4786, 20.3064)
  line L602 (60.4786, 20.3064) -> (60.2706, 19.7644)
  line L603 (60.2706, 19.7644) -> (59.8219, 19.7412)
  line L604 (59.8219, 19.7412) -> (59.3786, 19.7343)
  line L605 (59.3786, 19.7343) -> (58.9413, 19.7444)
  line L606 (58.9413, 19.7444) -> (58.5107, 19.7727)
  line L607 (58.5107, 19.7727) -> (58.0879, 19.8208)
  line L608 (58.0879, 19.8208) -> (57.8798, 19.8532)
  line L609 (57.8798, 19.8532) -> (57.7767, 19.8717)
  line L610 (57.7767, 19.8717) -> (57.6743, 19.8919)
  line L611 (57.6743, 19.8919) -> (57.3451, 19.1525)
  line L612 (57.3451, 19.1525) -> (57.4286, 19.0899)
  line L613 (57.4286, 19.0899) -> (57.5113, 19.0256)
  line L614 (57.5113, 19.0256) -> (57.6746, 18.8927)
  line L615 (57.6746, 18.8927) -> (57.9933, 18.6106)
  line L616 (57.9933, 18.6106) -> (58.3025, 18.3096)
  line L617 (58.3025, 18.3096) -> (58.6026, 17.9913)
  line L618 (58.6026, 17.9913) -> (58.8941, 17.6573)
  line L619 (58.8941, 17.6573) -> (59.1771, 17.3084)
  line L620 (59.1771, 17.3084) -> (58.9135, 16.7911)
  line L621 (58.9135, 16.7911) -> (58.4649, 16.8149)
  line L622 (58.4649, 16.8149) -> (58.0233, 16.8544)
  line L623 (58.0233, 16.8544) -> (57.5894, 16.9101)
  line L624 (57.5894, 16.9101) -> (57.1642, 16.9833)
  line L625 (57.1642, 16.9833) -> (56.7486, 17.0754)
  line L626 (56.7486, 17.0754) -> (56.5451, 17.1293)
  line L627 (56.5451, 17.1293) -> (56.4445, 17.1585)
  line L628 (56.4445, 17.1585) -> (56.3447, 17.1892)
  line L629 (56.3447, 17.1892) -> (55.9401, 16.4883)
  line L630 (55.9401, 16.4883) -> (56.0166, 16.4173)
  line L631 (56.0166, 16.4173) -> (56.0921, 16.3448)
  line L632 (56.0921, 16.3448) -> (56.2406, 16.1955)
  line L633 (56.2406, 16.1955) -> (56.5282, 15.8817)
  line L634 (56.5282, 15.8817) -> (56.8041, 15.55)
  line L635 (56.8041, 15.55) -> (57.0693, 15.2021)
  line L636 (57.0693, 15.2021) -> (57.3243, 14.8394)
  line L637 (57.3243, 14.8394) -> (57.5693, 14.4628)
  line L638 (57.5693, 14.4628) -> (57.2531, 13.9759)
  line L639 (57.2531, 13.9759) -> (56.8094, 14.0465)
  line L640 (56.8094, 14.0465) -> (56.3743, 14.1319)
  line L641 (56.3743, 14.1319) -> (55.9487, 14.2327)
  line L642 (55.9487, 14.2327) -> (55.5334, 14.3499)
  line L643 (55.5334, 14.3499) -> (55.1298, 14.4849)
  line L644 (55.1298, 14.4849) -> (54.933, 14.5599)
  line L645 (54.933, 14.5599) -> (54.836, 14.5994)
  line L646 (54.836, 14.5994) -> (54.74, 14.6404)
  line L647 (54.74, 14.6404) -> (54.2643, 13.9856)
  line L648 (54.2643, 13.9856) -> (54.3329, 13.907)
  line L649 (54.3329, 13.907) -> (54.4005, 13.827)
  line L650 (54.4005, 13.827) -> (54.5326, 13.663)
  line L651 (54.5326, 13.663) -> (54.7857, 13.3208)
  line L652 (54.7857, 13.3208) -> (55.0255, 12.9621)
  line L653 (55.0255, 12.9621) -> (55.2529, 12.5884)
  line L654 (55.2529, 12.5884) -> (55.4686, 12.201)
  line L655 (55.4686, 12.201) -> (55.6728, 11.8009)
  line L656 (55.6728, 11.8009) -> (55.3075, 11.3497)
  line L657 (55.3075, 11.3497) -> (54.8736, 11.4663)
  line L658 (54.8736, 11.4663) -> (54.4499, 11.5967)
  line L659 (54.4499, 11.5967) -> (54.0371, 11.7415)
  line L660 (54.0371, 11.7415) -> (53.6363, 11.9014)
  line L661 (53.6363, 11.9014) -> (53.249, 12.0779)
  line L662 (53.249, 12.0779) -> (53.0611, 12.173)
  line L663 (53.0611, 12.173) -> (52.9688, 12.2224)
  line L664 (52.9688, 12.2224) -> (52.8776, 12.2732)
  line L665 (52.8776, 12.2732) -> (52.3361, 11.6718)
  line L666 (52.3361, 11.6718) -> (52.3961, 11.5864)
  line L667 (52.3961, 11.5864) -> (52.455, 11.4998)
  line L668 (52.455, 11.4998) -> (52.5692, 11.3228)
  line L669 (52.5692, 11.3228) -> (52.7852, 10.9561)
  line L670 (52.7852, 10.9561) -> (52.9861, 10.5743)
  line L671 (52.9861, 10.5743) -> (53.1732, 10.1789)
  line L672 (53.1732, 10.1789) -> (53.3472, 9.7711)
  line L673 (53.3472, 9.7711) -> (53.5086, 9.3518)
  line L674 (53.5086, 9.3518) -> (53.098, 8.9413)
  line L675 (53.098, 8.9413) -> (52.6787, 9.1026)
  line L676 (52.6787, 9.1026) -> (52.2709, 9.2766)
  line L677 (52.2709, 9.2766) -> (51.8755, 9.4637)
  line L678 (51.8755, 9.4637) -> (51.4937, 9.6646)
  line L679 (51.4937, 9.6646) -> (51.127, 9.8806)
  line L680 (51.127, 9.8806) -> (50.9501, 9.9948)
  line L681 (50.9501, 9.9948) -> (50.8634, 10.0537)
  line L682 (50.8634, 10.0537) -> (50.778, 10.1137)
  line L683 (50.778, 10.1137) -> (50.1766, 9.5722)
  line L684 (50.1766, 9.5722) -> (50.2274, 9.481)
  line L685 (50.2274, 9.481) -> (50.2768, 9.3887)
  line L686 (50.2768, 9.3887) -> (50.3719, 9.2008)
  line L687 (50.3719, 9.2008) -> (50.5484, 8.8135)
  line L688 (50.5484, 8.8135) -> (50.7084, 8.4127)
  line L689 (50.7084, 8.4127) -> (50.8531, 7.9999)
  line L690 (50.8531, 7.9999) -> (50.9835, 7.5762)
  line L691 (50.9835, 7.5762) -> (51.1001, 7.1423)
  line L692 (51.1001, 7.1423) -> (50.6489, 6.777)
  line L693 (50.6489, 6.777) -> (50.2488, 6.9813)
  line L694 (50.2488, 6.9813) -> (49.8614, 7.1969)
  line L695 (49.8614, 7.1969) -> (49.4878, 7.4243)
  line L696 (49.4878, 7.4243) -> (49.129, 7.6641)
  line L697 (49.129, 7.6641) -> (48.7869, 7.9172)
  line L698 (48.7869, 7.9172) -> (48.6228, 8.0493)
  line L699 (48.6228, 8.0493) -> (48.5428, 8.1169)
  line L700 (48.5428, 8.1169) -> (48.4642, 8.1855)
  line L701 (48.4642, 8.1855) -> (47.8094, 7.7098)
  line L702 (47.8094, 7.7098) -> (47.8504, 7.6138)
  line L703 (47.8504, 7.6138) -> (47.8899, 7.5168)
  line L704 (47.8899, 7.5168) -> (47.9649, 7.32)
  line L705 (47.9649, 7.32) -> (48.0999, 6.9164)
  line L706 (48.0999, 6.9164) -> (48.2171, 6.5011)
  line L707 (48.2171, 6.5011) -> (48.3179, 6.0755)
  line L708 (48.3179, 6.0755) -> (48.4033, 5.6404)
  line L709 (48.4033, 5.6404) -> (48.4739, 5.1967)
  line L710 (48.4739, 5.1967) -> (47.987, 4.8805)
  line L711 (47.987, 4.8805) -> (47.6104, 5.1255)
  line L712 (47.6104, 5.1255) -> (47.2477, 5.3805)
  line L713 (47.2477, 5.3805) -> (46.8999, 5.6457)
  line L714 (46.8999, 5.6457) -> (46.5681, 5.9217)
  line L715 (46.5681, 5.9217) -> (46.2543, 6.2092)
  line L716 (46.2543, 6.2092) -> (46.105, 6.3577)
  line L717 (46.105, 6.3577) -> (46.0325, 6.4333)
  line L718 (46.0325, 6.4333) -> (45.9615, 6.5097)
  line L719 (45.9615, 6.5097) -> (45.2606, 6.1051)
  line L720 (45.2606, 6.1051) -> (45.2913, 6.0053)
  line L721 (45.2913, 6.0053) -> (45.3205, 5.9047)
  line L722 (45.3205, 5.9047) -> (45.3744, 5.7012)
  line L723 (45.3744, 5.7012) -> (45.4666, 5.2857)
  line L724 (45.4666, 5.2857) -> (45.5397, 4.8604)
  line L725 (45.5397, 4.8604) -> (45.5954, 4.4265)
  line L726 (45.5954, 4.4265) -> (45.6349, 3.9849)
  line L727 (45.6349, 3.9849) -> (45.6588, 3.5363)
  line L728 (45.6588, 3.5363) -> (45.1414, 3.2727)
  line L729 (45.1414, 3.2727) -> (44.7925, 3.5558)
  line L730 (44.7925, 3.5558) -> (44.4585, 3.8472)
  line L731 (44.4585, 3.8472) -> (44.1402, 4.1474)
  line L732 (44.1402, 4.1474) -> (43.8392, 4.4565)
  line L733 (43.8392, 4.4565) -> (43.5572, 4.7752)
  line L734 (43.5572, 4.7752) -> (43.4242, 4.9385)
  line L735 (43.4242, 4.9385) -> (43.3599, 5.0212)
  line L736 (43.3599, 5.0212) -> (43.2973, 5.1047)
  line L737 (43.2973, 5.1047) -> (42.558, 4.7756)
  line L738 (42.558, 4.7756) -> (42.5781, 4.6731)
  line L739 (42.5781, 4.6731) -> (42.5966, 4.5701)
  line L740 (42.5966, 4.5701) -> (42.629, 4.362)
  line L741 (42.629, 4.362) -> (42.6771, 3.9391)
  line L742 (42.6771, 3.9391) -> (42.7054, 3.5085)
  line L743 (42.7054, 3.5085) -> (42.7155, 3.0712)
  line L744 (42.7155, 3.0712) -> (42.7086, 2.6279)
  line L745 (42.7086, 2.6279) -> (42.6854, 2.1792)
  line L746 (42.6854, 2.1792) -> (42.1434, 1.9712)
  line L747 (42.1434, 1.9712) -> (41.826, 2.2891)
  line L748 (41.826, 2.2891) -> (41.5242, 2.6139)
  line L749 (41.5242, 2.6139) -> (41.2391, 2.9457)
  line L750 (41.2391, 2.9457) -> (40.972, 3.2846)
  line L751 (40.972, 3.2846) -> (40.7249, 3.631)
  line L752 (40.7249, 3.631) -> (40.6097, 3.8074)
  line L753 (40.6097, 3.8074) -> (40.5544, 3.8963)
  line L754 (40.5544, 3.8963) -> (40.5009, 3.9859)
  line L755 (40.5009, 3.9859) -> (39.7312, 3.7358)
  line L756 (39.7312, 3.7358) -> (39.7405, 3.6319)
  line L757 (39.7405, 3.6319) -> (39.7481, 3.5274)
  line L758 (39.7481, 3.5274) -> (39.7586, 3.3171)
  line L759 (39.7586, 3.3171) -> (39.7623, 2.8915)
  line L760 (39.7623, 2.8915) -> (39.7454, 2.4603)
  line L761 (39.7454, 2.4603) -> (39.7097, 2.0243)
  line L762 (39.7097, 2.0243) -> (39.6565, 1.5842)
  line L763 (39.6565, 1.5842) -> (39.5866, 1.1404)
  line L764 (39.5866, 1.1404) -> (39.0258, 0.9901)
  line L765 (39.0258, 0.9901) -> (38.7433, 1.3395)
  line L766 (38.7433, 1.3395) -> (38.4772, 1.6941)
  line L767 (38.4772, 1.6941) -> (38.2283, 2.0538)
  line L768 (38.2283, 2.0538) -> (37.998, 2.4188)
  line L769 (37.998, 2.4188) -> (37.7885, 2.7892)
  line L770 (37.7885, 2.7892) -> (37.6924, 2.9766)
  line L771 (37.6924, 2.9766) -> (37.6467, 3.0708)
  line L772 (37.6467, 3.0708) -> (37.6028, 3.1655)
  line L773 (37.6028, 3.1655) -> (36.8112, 2.9973)
  line L774 (36.8112, 2.9973) -> (36.8096, 2.8929)
  line L775 (36.8096, 2.8929) -> (36.8062, 2.7882)
  line L776 (36.8062, 2.7882) -> (36.7946, 2.5779)
  line L777 (36.7946, 2.5779) -> (36.7538, 2.1543)
  line L778 (36.7538, 2.1543) -> (36.692, 1.7273)
  line L779 (36.692, 1.7273) -> (36.6109, 1.2974)
  line L780 (36.6109, 1.2974) -> (36.512, 0.8652)
  line L781 (36.512, 0.8652) -> (36.3961, 0.4312)
  line L782 (36.3961, 0.4312) -> (35.8226, 0.3404)
  line L783 (35.8226, 0.3404) -> (35.5783, 0.7173)
  line L784 (35.5783, 0.7173) -> (35.3506, 1.0978)
  line L785 (35.3506, 1.0978) -> (35.1407, 1.4816)
  line L786 (35.1407, 1.4816) -> (34.9499, 1.8686)
  line L787 (34.9499, 1.8686) -> (34.7802, 2.2589)
  line L788 (34.7802, 2.2589) -> (34.7042, 2.4553)
  line L789 (34.7042, 2.4553) -> (34.6686, 2.5538)
  line L790 (34.6686, 2.5538) -> (34.6349, 2.6526)
  line L791 (34.6349, 2.6526) -> (33.83, 2.568)
  line L792 (33.83, 2.568) -> (33.8175, 2.4644)
  line L793 (33.8175, 2.4644) -> (33.8032, 2.3606)
  line L794 (33.8032, 2.3606) -> (33.7697, 2.1527)
  line L795 (33.7697, 2.1527) -> (33.6849, 1.7356)
  line L796 (33.6849, 1.7356) -> (33.5787, 1.3174)
  line L797 (33.5787, 1.3174) -> (33.4531, 0.8983)
  line L798 (33.4531, 0.8983) -> (33.3096, 0.4789)
  line L799 (33.3096, 0.4789) -> (33.1489, 0.0593)
  line L800 (33.1489, 0.0593) -> (32.5691, 0.029)
  line L801 (32.5691, 0.029) -> (32.3655, 0.4294)
  line L802 (32.3655, 0.4294) -> (32.1789, 0.8316)
  line L803 (32.1789, 0.8316) -> (32.0102, 1.2352)
  line L804 (32.0102, 1.2352) -> (31.8609, 1.64)
  line L805 (31.8609, 1.64) -> (31.7329, 2.0459)
  line L806 (31.7329, 2.0459) -> (31.6779, 2.2492)
  line L807 (31.6779, 2.2492) -> (31.6528, 2.3509)
  line L808 (31.6528, 2.3509) -> (31.6296, 2.4527)
  line L809 (31.6296, 2.4527) -> (30.8203, 2.4527)
  line L810 (30.8203, 2.4527) -> (30.797, 2.3509)
  line L811 (30.797, 2.3509) -> (30.772, 2.2492)
  line L812 (30.772, 2.2492) -> (30.7169, 2.0459)
  line L813 (30.7169, 2.0459) -> (30.5889, 1.64)
  line L814 (30.5889, 1.64) -> (30.4396, 1.2352)
  line L815 (30.4396, 1.2352) -> (30.2709, 0.8316)
  line L816 (30.2709, 0.8316) -> (30.0843, 0.4294)
  line L817 (30.0843, 0.4294) -> (29.8807, 0.0289)
  line L818 (29.8807, 0.0289) -> (29.3009, 0.0593)
  line L819 (29.3009, 0.0593) -> (29.1403, 0.4789)
  line L820 (29.1403, 0.4789) -> (28.9967, 0.8983)
  line L821 (28.9967, 0.8983) -> (28.8711, 1.3174)
  line L822 (28.8711, 1.3174) -> (28.765, 1.7356)
  line L823 (28.765, 1.7356) -> (28.6801, 2.1527)
  line L824 (28.6801, 2.1527) -> (28.6466, 2.3606)
  line L825 (28.6466, 2.3606) -> (28.6323, 2.4644)
  line L826 (28.6323, 2.4644) -> (28.6198, 2.568)
  line L827 (28.6198, 2.568) -> (27.8149, 2.6526)
  line L828 (27.8149, 2.6526) -> (27.7812, 2.5538)
  line L829 (27.7812, 2.5538) -> (27.7456, 2.4553)
  line L830 (27.7456, 2.4553) -> (27.6697, 2.2589)
  line L831 (27.6697, 2.2589) -> (27.4999, 1.8686)
  line L832 (27.4999, 1.8686) -> (27.3091, 1.4816)
  line L833 (27.3091, 1.4816) -> (27.0992, 1.0978)
  line L834 (27.0992, 1.0978) -> (26.8716, 0.7173)
  line L835 (26.8716, 0.7173) -> (26.6272, 0.3404)
  line L836 (26.6272, 0.3404) -> (26.0538, 0.4312)
  line L837 (26.0538, 0.4312) -> (25.9378, 0.8652)
  line L838 (25.9378, 0.8652) -> (25.8389, 1.2974)
  line L839 (25.8389, 1.2974) -> (25.7578, 1.7273)
  line L840 (25.7578, 1.7273) -> (25.696, 2.1543)
  line L841 (25.696, 2.1543) -> (25.6552, 2.5779)
  line L842 (25.6552, 2.5779) -> (25.6436, 2.7882)
  line L843 (25.6436, 2.7882) -> (25.6402, 2.8929)
  line L844 (25.6402, 2.8929) -> (25.6386, 2.9973)
  line L845 (25.6386, 2.9973) -> (24.847, 3.1655)
  line L846 (24.847, 3.1655) -> (24.8031, 3.0708)
  line L847 (24.8031, 3.0708) -> (24.7575, 2.9766)
  line L848 (24.7575, 2.9766) -> (24.6613, 2.7892)
  line L849 (24.6613, 2.7892) -> (24.4518, 2.4188)
  line L850 (24.4518, 2.4188) -> (24.2216, 2.0538)
  line L851 (24.2216, 2.0538) -> (23.9727, 1.6941)
  line L852 (23.9727, 1.6941) -> (23.7065, 1.3395)
  line L853 (23.7065, 1.3395) -> (23.4241, 0.9901)
  line L854 (23.4241, 0.9901) -> (22.8633, 1.1404)
  line L855 (22.8633, 1.1404) -> (22.7933, 1.5842)
  line L856 (22.7933, 1.5842) -> (22.7401, 2.0243)
  line L857 (22.7401, 2.0243) -> (22.7045, 2.4603)
  line L858 (22.7045, 2.4603) -> (22.6876, 2.8915)
  line L859 (22.6876, 2.8915) -> (22.6913, 3.3171)
  line L860 (22.6913, 3.3171) -> (22.7017, 3.5274)
  line L861 (22.7017, 3.5274) -> (22.7093, 3.6319)
  line L862 (22.7093, 3.6319) -> (22.7186, 3.7358)
  line L863 (22.7186, 3.7358) -> (21.949, 3.9859)
  line L864 (21.949, 3.9859) -> (21.8954, 3.8963)
  line L865 (21.8954, 3.8963) -> (21.8401, 3.8074)
  line L866 (21.8401, 3.8074) -> (21.725, 3.631)
  line L867 (21.725, 3.631) -> (21.4778, 3.2846)
  line L868 (21.4778, 3.2846) -> (21.2107, 2.9457)
  line L869 (21.2107, 2.9457) -> (20.9256, 2.6139)
  line L870 (20.9256, 2.6139) -> (20.6238, 2.2891)
  line L871 (20.6238, 2.2891) -> (20.3064, 1.9712)
  line L872 (20.3064, 1.9712) -> (19.7644, 2.1792)
  line L873 (19.7644, 2.1792) -> (19.7412, 2.6279)
  line L874 (19.7412, 2.6279) -> (19.7343, 3.0712)
  line L875 (19.7343, 3.0712) -> (19.7444, 3.5085)
  line L876 (19.7444, 3.5085) -> (19.7727, 3.9391)
  line L877 (19.7727, 3.9391) -> (19.8208, 4.362)
  line L878 (19.8208, 4.362) -> (19.8532, 4.5701)
  line L879 (19.8532, 4.5701) -> (19.8717, 4.6731)
  line L880 (19.8717, 4.6731) -> (19.8919, 4.7756)
  line L881 (19.8919, 4.7756) -> (19.1525, 5.1047)
  line L882 (19.1525, 5.1047) -> (19.0899, 5.0212)
  line L883 (19.0899, 5.0212) -> (19.0256, 4.9385)
  line L884 (19.0256, 4.9385) -> (18.8927, 4.7752)
  line L885 (18.8927, 4.7752) -> (18.6106, 4.4565)
  line L886 (18.6106, 4.4565) -> (18.3096, 4.1474)
  line L887 (18.3096, 4.1474) -> (17.9913, 3.8472)
  line L888 (17.9913, 3.8472) -> (17.6573, 3.5558)
  line L889 (17.6573, 3.5558) -> (17.3084, 3.2727)
  line L890 (17.3084, 3.2727) -> (16.7911, 3.5363)
  line L891 (16.7911, 3.5363) -> (16.8149, 3.9849)
  line L892 (16.8149, 3.9849) -> (16.8544, 4.4265)
  line L893 (16.8544, 4.4265) -> (16.9101, 4.8604)
  line L894 (16.9101, 4.8604) -> (16.9833, 5.2857)
  line L895 (16.9833, 5.2857) -> (17.0754, 5.7012)
  line L896 (17.0754, 5.7012) -> (17.1293, 5.9047)
  line L897 (17.1293, 5.9047) -> (17.1585, 6.0053)
  line L898 (17.1585, 6.0053) -> (17.1892, 6.1051)
  line L899 (17.1892, 6.1051) -> (16.4883, 6.5097)
  line L900 (16.4883, 6.5097) -> (16.4173, 6.4333)
  line L901 (16.4173, 6.4333) -> (16.3448, 6.3577)
  line L902 (16.3448, 6.3577) -> (16.1955, 6.2092)
  line L903 (16.1955, 6.2092) -> (15.8817, 5.9217)
  line L904 (15.8817, 5.9217) -> (15.55, 5.6457)
  line L905 (15.55, 5.6457) -> (15.2021, 5.3805)
  line L906 (15.2021, 5.3805) -> (14.8394, 5.1255)
  line L907 (14.8394, 5.1255) -> (14.4628, 4.8805)
  line L908 (14.4628, 4.8805) -> (13.9759, 5.1967)
  line L909 (13.9759, 5.1967) -> (14.0465, 5.6404)
  line L910 (14.0465, 5.6404) -> (14.1319, 6.0755)
  line L911 (14.1319, 6.0755) -> (14.2327, 6.5011)
  line L912 (14.2327, 6.5011) -> (14.3499, 6.9164)
  line L913 (14.3499, 6.9164) -> (14.4849, 7.32)
  line L914 (14.4849, 7.32) -> (14.5599, 7.5168)
  line L915 (14.5599, 7.5168) -> (14.5994, 7.6138)
  line L916 (14.5994, 7.6138) -> (14.6404, 7.7098)
  line L917 (14.6404, 7.7098) -> (13.9856, 8.1855)
  line L918 (13.9856, 8.1855) -> (13.907, 8.1169)
  line L919 (13.907, 8.1169) -> (13.827, 8.0493)
  line L920 (13.827, 8.0493) -> (13.663, 7.9172)
  line L921 (13.663, 7.9172) -> (13.3208, 7.6641)
  line L922 (13.3208, 7.6641) -> (12.9621, 7.4243)
  line L923 (12.9621, 7.4243) -> (12.5884, 7.1969)
  line L924 (12.5884, 7.1969) -> (12.201, 6.9813)
  line L925 (12.201, 6.9813) -> (11.8009, 6.777)
  line L926 (11.8009, 6.777) -> (11.3497, 7.1423)
  line L927 (11.3497, 7.1423) -> (11.4663, 7.5762)
  line L928 (11.4663, 7.5762) -> (11.5967, 7.9999)
  line L929 (11.5967, 7.9999) -> (11.7415, 8.4127)
  line L930 (11.7415, 8.4127) -> (11.9014, 8.8135)
  line L931 (11.9014, 8.8135) -> (12.0779, 9.2008)
  line L932 (12.0779, 9.2008) -> (12.173, 9.3887)
  line L933 (12.173, 9.3887) -> (12.2224, 9.481)
  line L934 (12.2224, 9.481) -> (12.2732, 9.5722)
  line L935 (12.2732, 9.5722) -> (11.6718, 10.1137)
  line L936 (11.6718, 10.1137) -> (11.5864, 10.0537)
  line L937 (11.5864, 10.0537) -> (11.4998, 9.9948)
  line L938 (11.4998, 9.9948) -> (11.3228, 9.8806)
  line L939 (11.3228, 9.8806) -> (10.9561, 9.6646)
  line L940 (10.9561, 9.6646) -> (10.5743, 9.4637)
  line L941 (10.5743, 9.4637) -> (10.1789, 9.2766)
  line L942 (10.1789, 9.2766) -> (9.7711, 9.1026)
  line L943 (9.7711, 9.1026) -> (9.3518, 8.9413)
  line L944 (9.3518, 8.9413) -> (8.9413, 9.3518)
  line L945 (8.9413, 9.3518) -> (9.1026, 9.7711)
  line L946 (9.1026, 9.7711) -> (9.2766, 10.1789)
  line L947 (9.2766, 10.1789) -> (9.4637, 10.5743)
  line L948 (9.4637, 10.5743) -> (9.6646, 10.9561)
  line L949 (9.6646, 10.9561) -> (9.8806, 11.3228)
  line L950 (9.8806, 11.3228) -> (9.9948, 11.4998)
  line L951 (9.9948, 11.4998) -> (10.0537, 11.5864)
  line L952 (10.0537, 11.5864) -> (10.1137, 11.6718)
  line L953 (10.1137, 11.6718) -> (9.5722, 12.2732)
  line L954 (9.5722, 12.2732) -> (9.481, 12.2224)